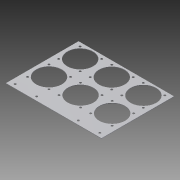
# Autodesk Inventor part: plate
Saved by Autodesk Inventor 2014 SP1 (Build 180222100, 222)
## iProperties
Created: 2016-09-05
Part Number: plate
Material: ABS Plastic
Document SubType Name: Modeling
Designer: tguillod
Density: 1.06 g/cm^3
Appearance: Smooth - White
Author: tguillod
Autodesk Inventor part; units mm, degrees
ref_plane "YZ Plane" through (0, 0, 0) normal (1, 0, 0) x (0, 1, 0)
ref_plane "XZ Plane" through (0, 0, 0) normal (0, 1, 0) x (-1, 0, 0)
ref_plane "XY Plane" through (0, 0, 0) normal (0, 0, 1) x (1, 0, 0)
sketch "Sketch1" plane through (0, 0, 0) normal (0, 0, 1) x (1, 0, 0)
  line L0 (0, 0) -> (177.5, 0)
  line L1 (177.5, 0) -> (177.5, 135)
  line L2 (177.5, 135) -> (0, 135)
  line L3 (0, 135) -> (0, 0)
  dimension "d0" = 177.5
  dimension "d1" = 135
  constraints: 8 end point, 2 parallel, 1 horizontal, 1 perpendicular
  measures "d0" distance of L1.end L2.end
  measures "d1" distance of L0.end L1.end
extrude "Extrusion1" add sketch "Sketch1" along normal blind 1
sketch "Sketch3" plane through (0, 0, 1) normal (0, 0, 1) x (1, 0, 0)
  line L0 (0, 0) -> (177.5, 0) projected
  line L1 (177.5, 0) -> (177.5, 135) projected
  line L2 (177.5, 135) -> (0, 135) projected
  line L3 (0, 135) -> (0, 0) projected
  line L4 (0, 128) -> (177.5, 128) construction
  line L5 (10, 135) -> (10, 0) construction
  line L6 (0, 88) -> (177.5, 88) construction
  line L7 (177.5, 70) -> (0, 70) construction
  line L8 (0, 30) -> (177.5, 30) construction
  line L9 (50, 135) -> (50, 0) construction
  line L10 (127.5, 135) -> (127.5, 0) construction
  line L11 (108.75, 135) -> (108.75, 0) construction
  line L12 (68.75, 135) -> (68.75, 0) construction
  line L13 (167.5, 135) -> (167.5, 0) construction
  line L14 (0, 7) -> (177.5, 7) construction
  point P0 (10, 128)
  point P1 (50, 128)
  point P2 (68.75, 128)
  point P3 (108.75, 128)
  point P4 (127.5, 128)
  point P5 (167.5, 128)
  point P6 (167.5, 88)
  point P7 (127.5, 88)
  point P8 (108.75, 88)
  point P9 (68.75, 88)
  point P10 (50, 88)
  point P11 (10, 88)
  point P12 (50, 30)
  point P13 (50, 70)
  point P14 (10, 70)
  point P15 (10, 30)
  point P16 (127.5, 30)
  point P17 (167.5, 30)
  point P18 (167.5, 70)
  point P19 (127.5, 70)
  point P20 (68.75, 70)
  point P21 (108.75, 70)
  point P22 (108.75, 30)
  point P23 (68.75, 30)
  point P24 (10, 7)
  point P25 (167.5, 7)
  point P26 (50, 7)
  point P27 (127.5, 7)
  dimension "d5" = 40
  dimension "d6" = 40
  dimension "d7" = 40
  dimension "d8" = 40
  dimension "d9" = 40
  dimension "d10" = 10
  dimension "d11" = 10
  dimension "d12" = 7
  dimension "d13" = 18
  dimension "d14" = 18.75
  dimension "d30" = 18.75
  dimension "d40" = 7
  constraints: 78 point on line, 22 end point, 9 perpendicular, 2 parallel
  measures "d5" distance between parallel lines of L9 L5
  measures "d6" distance between parallel lines of L6 L4
  measures "d7" distance between parallel lines of L8 L7
  measures "d8" distance between parallel lines of L11 L12
  measures "d9" distance between parallel lines of L13 L10
  measures "d10" distance between parallel lines of L5 L3
  measures "d11" distance between parallel lines of L1 L13
  measures "d12" distance between parallel lines of L4 L2
  measures "d13" distance between parallel lines of L7 L6
  measures "d14" distance between parallel lines of L12 L9
  measures "d30" distance between parallel lines of L10 L11
  measures "d40" distance between parallel lines of L14 L0
hole "Hole1" at (10, 128, 1) at (50, 128, 1) at (68.75, 128, 1) at (108.75, 128, 1) at (127.5, 128, 1) at (167.5, 128, 1) at (167.5, 88, 1) at (127.5, 88, 1) at (108.75, 88, 1) at (68.75, 88, 1) at (50, 88, 1) at (10, 88, 1) at (50, 30, 1) at (50, 70, 1) at (10, 70, 1) at (10, 30, 1) at (127.5, 30, 1) at (167.5, 30, 1) at (167.5, 70, 1) at (127.5, 70, 1) at (68.75, 70, 1) at (108.75, 70, 1) at (68.75, 30, 1) at (108.75, 30, 1) at (10, 7, 1) at (50, 7, 1) at (127.5, 7, 1) at (167.5, 7, 1) direction (0, 0, -1) diameter 4 end through all
sketch "Sketch4" plane through (0, 0, 1) normal (0, 0, 1) x (1, 0, 0)
  circle A0 centre (167.5, 70) radius 2 projected
  circle A1 centre (127.5, 30) radius 2 projected
  circle A2 centre (10, 70) radius 2 projected
  circle A3 centre (50, 30) radius 2 projected
  circle A4 centre (50, 88) radius 2 projected
  circle A5 centre (108.75, 88) radius 2 projected
  circle A6 centre (167.5, 88) radius 2 projected
  circle A7 centre (127.5, 128) radius 2 projected
  circle A8 centre (68.75, 128) radius 2 projected
  circle A9 centre (10, 128) radius 2 projected
  circle A10 centre (50, 128) radius 2 projected
  circle A11 centre (108.75, 128) radius 2 projected
  circle A12 centre (167.5, 128) radius 2 projected
  circle A13 centre (127.5, 88) radius 2 projected
  circle A14 centre (68.75, 88) radius 2 projected
  circle A15 centre (10, 88) radius 2 projected
  circle A16 centre (50, 70) radius 2 projected
  circle A17 centre (10, 30) radius 2 projected
  circle A18 centre (167.5, 30) radius 2 projected
  circle A19 centre (127.5, 70) radius 2 projected
  line L0 (10, 128) -> (50, 88) construction
  line L1 (68.75, 128) -> (108.75, 88) construction
  line L2 (50, 128) -> (10, 88) construction
  line L3 (68.75, 88) -> (108.75, 128) construction
  line L4 (127.5, 128) -> (167.5, 88) construction
  line L5 (167.5, 128) -> (127.5, 88) construction
  line L6 (127.5, 70) -> (167.5, 30) construction
  line L7 (167.5, 70) -> (127.5, 30) construction
  line L8 (10, 70) -> (50, 30) construction
  line L9 (50, 70) -> (10, 30) construction
  circle A20 centre (30, 108) radius 24
  circle A21 centre (88.75, 108) radius 24
  circle A22 centre (147.5, 108) radius 24
  circle A23 centre (147.5, 50) radius 24
  circle A24 centre (30, 50) radius 24
  circle A25 centre (68.75, 30) radius 2 projected
  circle A26 centre (68.75, 70) radius 2 projected
  circle A27 centre (108.75, 70) radius 2 projected
  circle A28 centre (108.75, 30) radius 2 projected
  line L10 (68.75, 70) -> (108.75, 30) construction
  line L11 (108.75, 70) -> (68.75, 30) construction
  circle A29 centre (88.75, 50) radius 24
  dimension "d22" = 48
  dimension "d23" = 48
  dimension "d24" = 48
  dimension "d25" = 48
  dimension "d26" = 48
  dimension "d29" = 48
  constraints: 24 end point, 9 perpendicular, 6 centre point, 6 midpoint, 2 parallel
  measures "d22" diameter of A20
  measures "d23" diameter of A21
  measures "d24" diameter of A22
  measures "d25" diameter of A23
  measures "d26" diameter of A24
  measures "d29" diameter of A29
extrude "Extrusion2" cut sketch "Sketch4" against normal blind 48 contours A20 | A21 | A22 | A23 | A24 | A29
equation "\"d27\" = d29"
body "Solid1"
